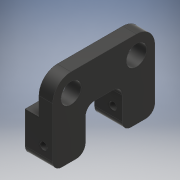
# Autodesk Inventor part: +XPanel_AntennaMount
Saved by Autodesk Inventor 2018 (Build 220112000, 112)
## iProperties
Created: 2018-07-06
Part Number: +XPanel_AntennaMount
Material: Acetal Resin, Black
Document SubType Name: Modeling
Designer: Bradley
Density: 1.425 g/cm^3
Appearance: Smooth - Black
Mass: 0.242096 g
Surface Area: 3.11902 cm^2
Volume: 0.169892 cm^3
Author: Bradley
Autodesk Inventor part; units mm, degrees
ref_plane "YZ Plane" through (0, 0, 0) normal (1, 0, 0) x (0, 1, 0)
ref_plane "XZ Plane" through (0, 0, 0) normal (0, 1, 0) x (-1, 0, 0)
ref_plane "XY Plane" through (0, 0, 0) normal (0, 0, 1) x (1, 0, 0)
sketch "Sketch1" plane through (0, 0, 0) normal (1, 0, 0) x (0, 1, 0)
  line L0 (-5.5714, 4.25) -> (5.5714, 4.25)
  line L1 (5.5714, 4.25) -> (5.5714, -4.25)
  line L2 (5.5714, -4.25) -> (-5.5714, -4.25)
  line L3 (-5.5714, -4.25) -> (-5.5714, 4.25)
  line L4 (-5.5714, 0.25) -> (5.5714, 0.25) construction
  circle A0 centre (-3.5714, 2.25) radius 2 construction
  line L5 (-2, -4.25) -> (2, -4.25)
  line L6 (2, -4.25) -> (2, 0.25)
  line L7 (2, 0.25) -> (-2, 0.25)
  line L8 (-2, 0.25) -> (-2, -4.25)
  circle A1 centre (3.5714, 2.25) radius 2 construction
  circle A2 centre (0, 36.35) radius 39 construction
  line L9 (-5.5714, -2.25) -> (5.5714, -2.25) construction
  point P0 (0, 0)
  point P1 (-5.5714, 0)
  point P2 (0, -4.25)
  dimension "d0" = 4
  dimension "d1" = 4.5
  dimension "d2" = 11.1427
  dimension "d15" = 4
  dimension "d34" = 78
  dimension "d35" = 38.6
  dimension "d36" = 4.5
  constraints: 20 end point, 6 point on line, 6 tangent, 4 horizontal, 4 parallel, 3 centre point, 3 midpoint, 2 perpendicular, 2 point on circle, 1 horizontal alignment, 1 vertical alignment
  measures "d0" diameter of A0
  measures "d1" distance between parallel lines of L2 L4
  measures "d2" distance of L0.start L0.end
  measures "d15" distance of L5.start L5.end
  measures "d34" diameter of A2
  measures "d35" distance from line of A2.centre L9
  measures "d36" distance from line of L9 A0.centre
extrude "Extrusion1" add sketch "Sketch1" along normal mid plane 3 contours L0 L1 L2 L6 L7 L8 L3
sketch "Sketch4" plane through (-1.5, -5.5714, -4.25) normal (0, -1, 0) x (1, 0, 0)
  line L0 (0, 8.5) -> (3, 8.5) projected
  line L1 (0, 0) -> (0, 8.5) projected
  line L2 (3, 0) -> (0, 0) projected
  line L3 (3, 8.5) -> (3, 0) projected
  circle A0 centre (2, 2) radius 0.3962
  point P0 (1.5, 4.25)
  dimension "d16" = 0.7925
  dimension "d24" = 2
  dimension "d25" = 6.5
  constraints: 1 centre point
  measures "d16" diameter of A0
  measures "d24" distance from line of L1 A0.centre
  measures "d25" distance from line of A0.centre L0
extrude "Extrusion3" cut sketch "Sketch4" against normal through all contours A0
fillet "Fillet1" radius 1 6 edges at (0, 2, 0.25) (0, -2, 0.25) (0, 2, -4.25) (0, -2, -4.25) (0, 5.5714, -4.25) (0, -5.5714, -4.25)
fillet "Fillet1" radius 2 2 edges at (0, 5.5714, 4.25) (0, -5.5714, 4.25)
sketch "Sketch5" plane through (-1.5, 0, 0) normal (-1, 0, 0) x (0, 0, 1)
  line L0 (-0.75, -2) -> (-3.25, -2) projected
  line L1 (-4.25, -3) -> (-4.25, -4.5714) projected
  line L2 (-3.25, -5.5714) -> (2.25, -5.5714) projected
  line L3 (4.25, -3.5714) -> (4.25, 3.5714) projected
  line L4 (2.25, 5.5714) -> (-3.25, 5.5714) projected
  line L5 (-4.25, 4.5714) -> (-4.25, 3) projected
  line L6 (-3.25, 2) -> (-0.75, 2) projected
  arc A0 (0.25, 1) -> (-0.75, 2) centre (-0.75, 1) ccw projected
  line L7 (0.25, 1) -> (0.25, -1) projected
  arc A1 (-0.75, -2) -> (0.25, -1) centre (-0.75, -1) ccw projected
  line L8 (-0.75, -2) -> (-3.25, -2) projected
  line L9 (-0.75, -2) -> (0.25, -2)
  arc A2 (-0.75, -2) -> (0.25, -1) centre (-0.75, -1) ccw projected
  line L10 (0.25, -2) -> (0.25, -5.5714)
  line L11 (-0.75, 2) -> (0.25, 2)
  line L12 (0.25, 2) -> (0.25, 5.5714)
  line L13 (2.25, 5.5714) -> (-3.25, 5.5714) projected
  line L14 (0.25, 1) -> (0.25, -1) projected
  arc A3 (4.25, 3.5714) -> (2.25, 5.5714) centre (2.25, 3.5714) ccw projected
  arc A4 (2.25, -5.5714) -> (4.25, -3.5714) centre (2.25, -3.5714) ccw projected
  arc A5 (-3.25, 5.5714) -> (-4.25, 4.5714) centre (-3.25, 4.5714) ccw projected
  arc A6 (-4.25, 3) -> (-3.25, 2) centre (-3.25, 3) ccw projected
  arc A7 (-3.25, -2) -> (-4.25, -3) centre (-3.25, -3) ccw projected
  arc A8 (-4.25, -4.5714) -> (-3.25, -5.5714) centre (-3.25, -4.5714) ccw projected
  point P0 (0, 0)
  point P1 (4.25, 7)
  point P2 (-4.25, 7)
  constraints: 8 end point, 3 point on line, 2 perpendicular, 1 collinear, 1 horizontal, 1 tangent, 2 other
extrude "Extrusion4" cut sketch "Sketch5" against normal blind 1.5 contours A1 L7 A0 L11 L12 L4 A3 L3 A4 L2 L10 L9
hole "Hole2" at (0, -3.5714, 2.25) at (0, 3.5714, 2.25) direction (1, 0, 0) diameter 2.2 end through all clearance for "Flat Head Machine Screw" size "M2" standard "Ansi Metric M Profile"
body "Solid1"
